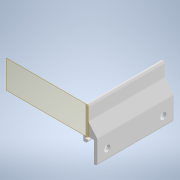
# Autodesk Inventor part: BackPistonSupportButtom
Saved by Autodesk Inventor 2022 (Build 260153000, 153)
## iProperties
Created: 2022-02-16
Part Number: BackPistonSupportButtom
Material: Generic
Document SubType Name: Modeling
Designer: siwat
Density: 1 g/cm^3
Appearance: Default
VLDS_Profile: Default Part
VLDS_TimeStamp: 2022-03-14
VLDS_FailCnt: 1
VLDS_AcceptCnt: 0
Author: siwat
Autodesk Inventor part; units mm, degrees
ref_plane "YZ Plane" through (0, 0, 0) normal (1, 0, 0) x (0, 1, 0)
ref_plane "XZ Plane" through (0, 0, 0) normal (0, 1, 0) x (-1, 0, 0)
ref_plane "XY Plane" through (0, 0, 0) normal (0, 0, 1) x (1, 0, 0)
ref_plane "Work Plane1" through (0, 0, 0) normal (0, 0, 1) x (1, 0, 0)
sketch "Sketch1" plane through (0, 0, 0) normal (0, 0, 1) x (1, 0, 0)
  line L0 (40.3399, -2.3219) -> (40.3399, -3.3134)
  line L1 (40.3399, -3.3134) -> (38.2935, -5.4505)
  line L2 (38.2935, -5.4505) -> (35.4492, -5.4505)
  line L3 (35.4492, -5.4505) -> (35.4492, -0.1275)
  line L4 (35.4492, -0.1275) -> (37.5466, -0.1275)
  line L5 (37.5466, -0.1275) -> (37.5466, 27.0272)
  line L6 (37.5466, 27.0272) -> (40.3399, 27.0272)
  line L7 (40.3399, 27.0272) -> (40.3399, 0.5164)
  line L8 (40.3399, 0.5164) -> (39.7973, 0.5164)
  line L9 (39.7973, 0.5164) -> (37.8585, -1.5084)
  line L10 (37.8585, -1.5084) -> (37.0796, -2.3219)
  line L11 (37.0796, -2.3219) -> (40.3399, -2.3219)
  line L12 (40.3399, 3.1566) -> (48.9527, 3.1566)
  line L13 (48.9527, 3.1566) -> (48.9527, -20.1251)
  line L14 (48.9527, -20.1251) -> (45.6975, -20.1251)
  line L15 (45.6975, -20.1251) -> (45.6975, 0.5164)
  line L16 (45.6975, 0.5164) -> (40.3399, 0.5164)
  point P0 (0, 0)
  dimension "d13" = 20.1251
  constraints: 34 end point, 10 perpendicular, 4 point on line, 2 parallel, 1 horizontal, 1 vertical
  measures "d13" distance from line of point (0, 0) L14
extrude "Extrusion1" add sketch "Sketch1" against normal blind 75
draft "FaceDraft1" angle -50 pull direction (-1, 0, 0) faces at (46.0818, 3.1566, -50) fixed edges at (48.9527, 3.1566, -37.5)
sketch "Sketch2" plane through (48.9527, -20.1251, 0) normal (1, 0, 0) x (0, 0, -1)
  circle A0 centre (10, 10) radius 3
  circle A1 centre (65, 10) radius 3
  line L0 (10, 10) -> (65, 10)
  line L1 (0, 0) -> (0, 23.2817) projected
  line L2 (75, 23.2817) -> (75, 0) projected
  line L3 (0, 0) -> (75, 0) projected
  point P0 (0, 20.1251)
  dimension "d19" = 6
  dimension "d20" = 6
  dimension "d21" = 10
  dimension "d22" = 10
  dimension "d23" = 10
  constraints: 2 centre point, 2 end point, 1 horizontal
  measures "d19" diameter of A0
  measures "d20" diameter of A1
  measures "d21" distance from line of L0.start L1
  measures "d22" distance from line of L2 L0.end
  measures "d23" distance from line of L3 L0.start
extrude "Extrusion2" cut sketch "Sketch2" against normal through all
fillet "Fillet2" radius 2 4 edges at (48.9527, 3.1566, -37.5) (40.3399, 13.421, -37.5) (40.3399, 27.0272, -37.5) (48.9527, -20.1251, -37.5)
equation "\"d22\" = d21"
body "Solid1"
